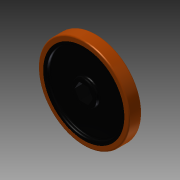
# Autodesk Inventor part: Wheel_73mm-10mm-HexMount_40A
Saved by Autodesk Inventor 2014 SP1 (Build 180222100, 222)
## iProperties
Created: 2015-04-11
Part Number: Wheel_73mm-10mm-HexMount_40A
Material: Rubber
Document SubType Name: Modeling
Designer: david
Density: 0.93 g/cm^3
Appearance: Smooth - Black
Mass: 23.5108 g
Surface Area: 157.844 cm^2
Volume: 25.2804 cm^3
Author: david
Autodesk Inventor part; units mm, degrees
ref_plane "YZ Plane" through (0, 0, 0) normal (1, 0, 0) x (0, 1, 0)
ref_plane "XZ Plane" through (0, 0, 0) normal (0, 1, 0) x (-1, 0, 0)
ref_plane "XY Plane" through (0, 0, 0) normal (0, 0, 1) x (1, 0, 0)
sketch "Sketch1" plane through (0, 0, 0) normal (0, 1, 0) x (-1, 0, 0)
  circle A0 centre (0, 0) radius 32.5
  line L0 (7.3323, 0) -> (3.6662, -6.35)
  line L1 (3.6662, -6.35) -> (-3.6662, -6.35)
  line L2 (-3.6662, -6.35) -> (-7.3323, 0)
  line L3 (-7.3323, 0) -> (-3.6662, 6.35)
  line L4 (-3.6662, 6.35) -> (3.6662, 6.35)
  line L5 (3.6662, 6.35) -> (7.3323, 0)
  dimension "d0" = 65
  dimension "d2" = 12.7
  constraints: 12 end point, 2 coincident, 1 centre point, 13 other
  measures "d0" diameter of A0
  measures "d2" distance between parallel lines of L1 L4
extrude "Extrusion1" add sketch "Sketch1" along normal blind 10
sketch "Sketch2" plane through (0, 10, 0) normal (0, 1, 0) x (1, 0, 0)
  circle A0 centre (0, 0) radius 32.5 projected
  circle A1 centre (0, 0) radius 36.5
  dimension "d5" = 73
  constraints: 1 centre point, 1 coincident
  measures "d5" diameter of A1
extrude "Extrusion2" add sketch "Sketch2" against normal blind 10 separate body
fillet "Fillet1" radius 0.5 6 edges at (-7.3323, 5, 0) (-3.6662, 5, -6.35) (3.6662, 5, -6.35) (7.3323, 5, 0) (3.6662, 5, 6.35) (-3.6662, 5, 6.35)
sketch "Sketch3" plane through (0, 10, 0) normal (0, 1, 0) x (1, 0, 0)
  circle A0 centre (0, 0) radius 32.5 projected
  circle A1 centre (0, 0) radius 10
  circle A2 centre (0, 0) radius 30
  dimension "d9" = 20
  dimension "d10" = 60
  constraints: 2 centre point, 2 coincident
  measures "d9" diameter of A1
  measures "d10" diameter of A2
extrude "Extrusion3" cut sketch "Sketch3" against normal blind 3 contours A2 bodies 1
sketch "Sketch4" plane through (0, 0, 0) normal (0, -1, 0) x (1, 0, 0)
  circle A0 centre (0, 0) radius 32.5 projected
  circle A1 centre (0, 0) radius 10
  circle A2 centre (0, 0) radius 30
  dimension "d13" = 20
  dimension "d14" = 60
  constraints: 2 centre point, 2 coincident
  measures "d13" diameter of A1
  measures "d14" diameter of A2
extrude "Extrusion4" cut sketch "Sketch4" against normal blind 3 contours A2 bodies 1
fillet "Fillet2" radius 1 10 edges at (-30, 3, 0) (-30, 0, 0) (-10, 3, 0) (-10, 0, 0) (-30, 10, 0) (-10, 10, 0) (-10, 7, 0) (-30, 7, 0) (-36.5, 0, 0) (-36.5, 10, 0)
body "Solid1"
body "Solid2"
